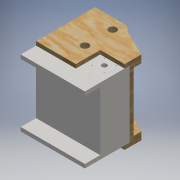
# Autodesk Inventor part: sideskirt_mount
Saved by Autodesk Inventor 2016 SP2 (Build 200236200, 236)
## iProperties
Created: 2017-08-25
Part Number: sideskirt_mount
Material: Generic
Document SubType Name: Modeling
Designer: Admin
Density: 1 g/cm^3
Appearance: Default
Tebal_papan: 15,000 mm
Lebar_base: 230,000 mm
box_nema23: 100,000 mm
d55: 145,251 mm
d60: 230,000 mm
d67: 100,000 mm
d70: 85,000 mm
d73: 230,000 mm
d80: 250,000 mm
d87: 230,000 mm
d94: 230,000 mm
d100: 70,000 mm
d106: 100,000 mm
d110: 230,000 mm
d113: 100,000 mm
d126: 360,00 deg
d0: 30,000 mm
d1: 30,000 mm
d2: 108,000 mm
d3: 150,000 mm
d5: 80,000 mm
d7: 15,000 mm
d8: 0,00 deg
d9: 15,000 mm
d10: 100,000 mm
d11: 100,000 mm
d12: 60,000 mm
d13: 15,000 mm
d14: 0,00 deg
d15: 230,000 mm
d16: 0,00 deg
d17: 80,000 mm
d32: 15,000 mm
d33: 15,000 mm
d34: 15,000 mm
d35: 230,000 mm
d36: 0,00 deg
d37: 230,000 mm
d38: 0,00 deg
d39: 230,000 mm
d40: 0,00 deg
d41: 15,000 mm
d42: 0,00 deg
d43: 15,000 mm
d44: 230,000 mm
d45: 0,00 deg
d46: 15,000 mm
d47: 230,000 mm
d48: 0,00 deg
d52: 15,000 mm
d53: 230,000 mm
d54: 0,00 deg
d56: 48,417 mm
d57: 48,417 mm
d58: 15,000 mm
d59: 0,00 deg
d61: 46,000 mm
d62: 46,000 mm
d63: 46,000 mm
d64: 46,000 mm
d65: 15,000 mm
d66: 0,00 deg
d68: 33,333 mm
d69: 33,333 mm
d71: 15,000 mm
d72: 42,500 mm
d74: 46,000 mm
d75: 46,000 mm
d76: 46,000 mm
d77: 46,000 mm
d78: 15,000 mm
d79: 0,00 deg
d81: 50,000 mm
d82: 50,000 mm
d83: 50,000 mm
d84: 50,000 mm
d85: 15,000 mm
d86: 0,00 deg
d88: 46,000 mm
d89: 46,000 mm
d90: 46,000 mm
d91: 46,000 mm
d92: 15,000 mm
d93: 0,00 deg
d95: 46,000 mm
d96: 46,000 mm
d97: 46,000 mm
d98: 46,000 mm
d99: 15,000 mm
d101: 23,333 mm
d102: 23,333 mm
d103: 15,000 mm
d104: 0,00 deg
d105: 15,000 mm
d107: 33,333 mm
d108: 33,333 mm
d109: 15,000 mm
d111: 32,857 mm
d112: 32,857 mm
d114: 33,333 mm
d115: 15,000 mm
d116: 0,00 deg
d117: 15,000 mm
d118: 15,000 mm
d120: 15,000 mm
d121: 0,00 deg
d122: 4,000 mm
d123: 23,570 mm
d124: 4,000 ul
d128: 20,000 mm
d129: 15,000 mm
d130: 0,00 deg
d131: 15,000 mm
d132: 250,000 mm
d133: 140,000 mm
d134: 95,000 mm
d135: 95,000 mm
Author: Admin
Autodesk Inventor part; units mm, degrees
ref_plane "YZ Plane" through (0, 0, 0) normal (1, 0, 0) x (0, 1, 0)
ref_plane "XZ Plane" through (0, 0, 0) normal (0, 1, 0) x (-1, 0, 0)
sketch "Sketch1" plane through (0, 0, 0) normal (0, 0, 1) x (1, 0, 0)
  circle A0 centre (0, 108) radius 15
  circle A1 centre (0, 0) radius 15
  line L0 (-110, 0) -> (-110, 150)
  line L1 (-110, 150) -> (0, 150)
  line L2 (140, 0) -> (140, -80)
  line L3 (140, -80) -> (0, -80)
  line L4 (-110, 0) -> (-110, -80)
  line L5 (-110, -80) -> (0, -80)
  circle A2 centre (0, 108) radius 42 construction
  arc A3 (35.2506, 130.834) -> (0, 150) centre (0, 108) ccw
  line L6 (140, 0) -> (140, 80)
  line L7 (35.2506, 130.834) -> (140, 80)
  dimension "d0" = 30
  dimension "d1" = 30
  dimension "d2" = 108
  dimension "d3" = 150
  dimension "d5" = 80
  dimension "d17" = 80
  dimension "d132" = 250
  dimension "d133" = 140
  constraints: 16 end point, 5 vertical alignment, 4 centre point, 4 point on circle, 4 vertical, 3 coincident, 3 perpendicular, 2 horizontal alignment
  measures "d0" diameter of A1
  measures "d1" diameter of A0
  measures "d2" distance of point (0, 0) A0.centre
  measures "d3" distance of L0.start L0.end
  measures "d5" distance of L2.start L2.end
  measures "d17" distance of L2.start L6.end
  measures "d132" distance of L4.end L2.end
  measures "d133" distance of L2.start point (0, 0)
extrude "Extrusion1" add sketch "Sketch1" along normal blind 15
sketch "Sketch2" plane through (0, 0, 15) normal (0, 0, 1) x (1, 0, 0)
  line L0 (140, -80) -> (140, 80.0243)
  line L1 (-110, 150) -> (-110, -80) projected
  line L2 (140, -65) -> (-110, -65)
  line L3 (-110, -65) -> (-110, -80)
  line L4 (-110, -80) -> (140, -80)
  line L5 (140, -80) -> (140, -65)
  line L6 (140, -65) -> (40, -65)
  line L7 (40, -65) -> (40, 35)
  line L8 (40, 35) -> (140, 35)
  line L9 (140, 35) -> (140, -65)
  line L10 (140, -80) -> (-110, -80) projected
  line L11 (140, -80) -> (-110, -80)
  line L12 (-110, -80) -> (-110, -140)
  line L13 (-110, -140) -> (140, -140)
  line L14 (140, -140) -> (140, -80)
  point P0 (0, 0)
  point P1 (120, 0)
  dimension "d9" = 15
  dimension "d10" = 100
  dimension "d11" = 100
  dimension "d12" = 60
  constraints: 24 end point, 5 parallel, 3 horizontal, 3 perpendicular, 2 vertical alignment, 1 vertical, 4 other
  measures "d9" distance of L1.end L2.end
  measures "d10" distance of L7.end L8.end
  measures "d11" distance of L6.end L7.end
  measures "d12" distance of L12.end L11.end
extrude "Extrusion2" add sketch "Sketch2" along normal blind 15 separate body
sketch "Sketch3" plane through (0, 0, 30) normal (0, 0, 1) x (1, 0, 0)
  line L0 (40, -65) -> (-110, -65) projected
  line L1 (-110, -80) -> (140, -80) projected
  line L2 (-110, -65) -> (140, -65)
  line L3 (140, -65) -> (140, -80)
  line L4 (140, -80) -> (-110, -80)
  line L5 (-110, -80) -> (-110, -65)
  point P0 (0, 0)
  constraints: 8 end point, 2 parallel, 1 horizontal, 1 perpendicular
extrude "Extrusion3" add sketch "Sketch3" along normal blind 230 separate body
sketch "Sketch5" plane through (0, 0, 30) normal (0, 0, 1) x (1, 0, 0)
  line L0 (40, 35) -> (40, -65) projected
  line L1 (140, 35) -> (40, 35) projected
  line L2 (140, -65) -> (-110, -65) projected
  line L3 (40, 35) -> (55, 35)
  line L4 (55, 35) -> (55, -65)
  line L5 (55, -65) -> (40, -65)
  line L6 (40, -65) -> (40, 35)
  point P0 (0, 0)
  dimension "d32" = 15
  constraints: 8 end point, 2 parallel, 1 horizontal, 1 perpendicular, 1 point on line
  measures "d32" distance of L4.end L5.end
sketch "Sketch6" plane through (0, 0, 30) normal (0, 0, 1) x (1, 0, 0)
  line L0 (140, -140) -> (140, 35) projected
  line L1 (140, 35) -> (40, 35) projected
  line L2 (140, -65) -> (-110, -65) projected
  line L3 (140, 35) -> (125, 35)
  line L4 (125, 35) -> (125, -65)
  line L5 (125, -65) -> (140, -65)
  line L6 (140, -65) -> (140, 35)
  point P0 (0, 0)
  dimension "d33" = 15
  constraints: 8 end point, 2 parallel, 1 horizontal, 1 perpendicular, 1 point on line
  measures "d33" distance of L5.end L4.end
sketch "Sketch7" plane through (0, 0, 30) normal (0, 0, 1) x (1, 0, 0)
  line L0 (140, 35) -> (40, 35) projected
  line L1 (55, 35) -> (125, 35)
  line L2 (55, 20) -> (125, 20)
  line L3 (55, 20) -> (55, 35)
  line L4 (125, 20) -> (125, 35)
  point P0 (0, 0)
  dimension "d34" = 15
  dimension "d117" = 15
  dimension "d118" = 15
  constraints: 8 end point, 2 point on line, 1 horizontal, 1 perpendicular, 1 vertical
  measures "d34" distance between parallel lines of L0 L2
  measures "d117" distance from line of L0.end L3
  measures "d118" distance of L0.start L1.end
extrude "Extrusion8" add sketch "Sketch5" along normal blind 230 separate body
extrude "Extrusion9" add sketch "Sketch7" along normal blind 230 separate body
extrude "Extrusion10" add sketch "Sketch6" along normal blind 230 separate body
sketch "Sketch8" plane through (0, 0, 15) normal (0, 0, 1) x (1, 0, 0)
  circle A0 centre (0, 0) radius 15 projected
  circle A1 centre (0, 108) radius 15 projected
  line L0 (-110, 150) -> (-110, -80) projected
  line L1 (-110, -80) -> (140, -80) projected
  line L2 (140, -80) -> (140, 80) projected
  line L3 (140, 80) -> (35.2506, 130.834) projected
  arc A2 (35.2506, 130.834) -> (0, 150) centre (0, 108) ccw projected
  line L4 (0, 150) -> (-110, 150) projected
  line L5 (125, 35) -> (55, 35) projected
  line L6 (140, 35) -> (125, 35) projected
  line L7 (55, 35) -> (40, 35) projected
  line L8 (40, 35) -> (40, -65) projected
  line L9 (40, -65) -> (-110, -65) projected
  line L10 (-110, 150) -> (-110, -80) projected
  line L11 (-110, 150) -> (-110, -65)
  line L12 (140, 35) -> (40, 35) projected
  line L13 (40, -65) -> (40, 35)
  line L14 (140, -140) -> (140, 35) projected
  line L15 (40, 35) -> (140, 35)
  constraints: 6 end point, 2 perpendicular, 1 vertical
extrude "Extrusion11" add sketch "Sketch8" along normal blind 15 separate body contours L4 A2 L3 L2 L6 L5 L7 L8 L9 L0
sketch "Sketch9" plane through (0, 0, 30) normal (0, 0, 1) x (1, 0, 0)
  line L0 (140, 35) -> (40, 35) projected
  line L1 (140, -80) -> (140, 80) projected
  line L2 (40, 35) -> (140, 35)
  line L3 (140, 35) -> (140, 50)
  line L4 (140, 50) -> (40, 50)
  line L5 (40, 50) -> (40, 35)
  point P0 (0, 0)
  dimension "d43" = 15
  constraints: 8 end point, 2 parallel, 1 horizontal, 1 perpendicular, 1 point on line
  measures "d43" distance of L3.end L2.end
extrude "Extrusion12" add sketch "Sketch9" along normal blind 230 separate body
sketch "Sketch10" plane through (0, 0, 30) normal (0, 0, 1) x (1, 0, 0)
  line L0 (140, -65) -> (-110, -65) projected
  line L1 (40, 35) -> (40, -65) projected
  line L2 (-110, -65) -> (40, -65)
  line L3 (40, -65) -> (40, -50)
  line L4 (40, -50) -> (-110, -50)
  line L5 (-110, -50) -> (-110, -65)
  point P0 (0, 0)
  dimension "d46" = 15
  constraints: 8 end point, 2 parallel, 1 horizontal, 1 perpendicular, 1 point on line
  measures "d46" distance of L3.end L2.end
extrude "Extrusion13" add sketch "Sketch10" along normal blind 230 separate body
sketch "Sketch12" plane through (0, 0, 30) normal (0, 0, 1) x (1, 0, 0)
  line L0 (140, 50) -> (40, 50) projected
  line L1 (40, -50) -> (-110, -50) projected
  line L2 (40, 50) -> (25, 50)
  line L3 (25, 50) -> (25, -50)
  line L4 (25, -50) -> (40, -50)
  line L5 (40, -50) -> (40, 50)
  point P0 (0, 0)
  dimension "d52" = 15
  constraints: 8 end point, 2 parallel, 1 horizontal, 1 perpendicular, 1 point on line
  measures "d52" distance of L4.end L3.end
extrude "Extrusion15" add sketch "Sketch12" along normal blind 230 separate body
sketch "Sketch13" plane through (-110, -50, 30) normal (0, 1, 0) x (1, 0, 0)
  line L0 (110, 0) -> (0, 0) projected
  line L1 (110, 0) -> (145.2506, 0) projected
  line L2 (0, 0) -> (250, 0) projected
  line L3 (150, 15) -> (0, 15) projected
  line L4 (0, 0) -> (48.4169, 0)
  line L5 (48.4169, 0) -> (48.4169, 15)
  line L6 (48.4169, 15) -> (0, 15)
  line L7 (0, 15) -> (0, 0)
  line L8 (145.2506, 0) -> (96.8338, 0)
  line L9 (96.8338, 0) -> (96.8338, 15)
  line L10 (96.8338, 15) -> (145.2506, 15)
  line L11 (145.2506, 15) -> (145.2506, 0)
  line L12 (0, 0) -> (0, -230) projected
  line L13 (0, 0) -> (0, -230) construction
  line L14 (0, -115) -> (68.0794, -115) construction
  line L15 (110, -230) -> (0, -230)
  line L16 (110, -230) -> (145.2506, -230)
  line L17 (150, -245) -> (0, -245)
  line L18 (0, -230) -> (48.4169, -230)
  line L19 (48.4169, -230) -> (48.4169, -245)
  line L20 (48.4169, -245) -> (0, -245)
  line L21 (0, -245) -> (0, -230)
  line L22 (145.2506, -230) -> (96.8338, -230)
  line L23 (96.8338, -230) -> (96.8338, -245)
  line L24 (96.8338, -245) -> (145.2506, -245)
  line L25 (145.2506, -245) -> (145.2506, -230)
  point P0 (110, 30)
  point P1 (110, -260)
  dimension "d55" = 145.2506
  dimension "d56" = 48.4169
  dimension "d57" = 48.4169
  constraints: 40 end point, 11 symmetric about line, 4 parallel, 4 point on line, 3 horizontal, 2 perpendicular, 1 midpoint
  measures "d55" distance of L1.end L0.end
  measures "d56" distance of L3.end L5.end
  measures "d57" distance of L10.end L9.end
extrude "Extrusion16" add sketch "Sketch13" against normal blind 15 contours L0 L9 L3 L11 L1 | L0 L7 L3 L5 | L16 L25 L17 L23 L15 | L19 L17 L21 L15 bodies 9
sketch "Sketch14" plane through (40, 50, 30) normal (0, 1, 0) x (1, 0, 0)
  line L0 (0, 0) -> (0, -230) projected
  line L1 (100, -230) -> (0, -230) projected
  line L2 (50, -230) -> (50, -65.4779) construction
  line L3 (-15, 0) -> (-15, -230) projected
  line L4 (0, 0) -> (-15, 0)
  line L5 (-15, 0) -> (-15, -46)
  line L6 (-15, -46) -> (0, -46)
  line L7 (0, -46) -> (0, 0)
  line L8 (0, 0) -> (0, -230) projected
  line L9 (0, -92) -> (-15, -92)
  line L10 (-15, -92) -> (-15, -138)
  line L11 (-15, -138) -> (0, -138)
  line L12 (0, -138) -> (0, -92)
  line L13 (0, -230) -> (-15, -230) projected
  line L14 (0, -230) -> (-15, -230)
  line L15 (-15, -230) -> (-15, -184)
  line L16 (-15, -184) -> (0, -184)
  line L17 (0, -184) -> (0, -230)
  line L18 (100, 15) -> (0, 15) projected
  line L19 (0, 0) -> (33.3333, 0)
  line L20 (33.3333, 0) -> (33.3333, 15)
  line L21 (33.3333, 15) -> (0, 15)
  line L22 (0, 15) -> (0, 0)
  line L23 (100, 0) -> (0, 0) projected
  line L24 (66.6667, 0) -> (100, 0)
  line L25 (100, 0) -> (100, 15)
  line L26 (100, 15) -> (66.6667, 15)
  line L27 (66.6667, 15) -> (66.6667, 0)
  line L28 (0, -115) -> (60, -115) construction
  line L29 (0, -230) -> (33.3333, -230)
  line L30 (33.3333, -230) -> (33.3333, -245)
  line L31 (33.3333, -245) -> (0, -245)
  line L32 (0, -245) -> (0, -230)
  line L33 (66.6667, -230) -> (100, -230)
  line L34 (100, -230) -> (100, -245)
  line L35 (100, -245) -> (66.6667, -245)
  line L36 (66.6667, -245) -> (66.6667, -230)
  point P0 (-40, 30)
  dimension "d60" = 230
  dimension "d61" = 46
  dimension "d62" = 46
  dimension "d63" = 46
  dimension "d64" = 46
  dimension "d67" = 100
  dimension "d68" = 33.3333
  dimension "d69" = 33.3333
  constraints: 60 end point, 10 parallel, 9 symmetric about line, 6 perpendicular, 6 point on line, 5 horizontal, 2 midpoint, 1 vertical
  measures "d60" distance of L0.end L0.start
  measures "d61" distance of L5.end L3.start
  measures "d62" distance of L9.end L5.end
  measures "d63" distance of L10.end L9.end
  measures "d64" distance of L3.end L15.end
  measures "d67" distance of L1.start L0.end
  measures "d68" distance of L20.end L18.end
  measures "d69" distance of L18.start L26.end
extrude "Extrusion17" add sketch "Sketch14" against normal blind 15 contours L1 L30 L31 L32 | L0 L6 L3 L4 | L22 L18 L20 L19 | L0 L11 L3 L9 | L27 L18 L25 L23 | L0 L13 L3 L16 | L34 L35 L36 L1 bodies 8
sketch "Sketch15" plane through (25, -50, 30) normal (-1, 0, 0) x (0, 0, 1)
  line L0 (230, 85) -> (184, 85) projected
  line L1 (230, 100) -> (230, 0) projected
  line L2 (230, 85) -> (245, 85)
  line L3 (245, 85) -> (245, 42.5)
  line L4 (245, 42.5) -> (230, 42.5)
  line L5 (230, 42.5) -> (230, 85)
  line L6 (0, 100) -> (230, 100) construction
  line L7 (115, 100) -> (115, 19.3986) construction
  line L8 (0, 85) -> (-15, 85)
  line L9 (-15, 85) -> (-15, 42.5)
  line L10 (-15, 42.5) -> (0, 42.5)
  line L11 (0, 42.5) -> (0, 85)
  line L12 (0, 0) -> (230, 0) construction
  line L13 (0, -15) -> (230, -15) projected
  line L14 (184, 0) -> (138, 0)
  line L15 (138, 0) -> (138, -15)
  line L16 (138, -15) -> (184, -15)
  line L17 (184, -15) -> (184, 0)
  line L18 (92, 0) -> (46, 0)
  line L19 (46, 0) -> (46, -15)
  line L20 (46, -15) -> (92, -15)
  line L21 (92, -15) -> (92, 0)
  point P0 (-30, 50)
  dimension "d70" = 85
  dimension "d71" = 15
  dimension "d72" = 42.5
  dimension "d73" = 230
  dimension "d74" = 46
  dimension "d75" = 46
  dimension "d76" = 46
  dimension "d77" = 46
  constraints: 34 end point, 6 parallel, 4 point on line, 4 symmetric about line, 3 horizontal, 3 perpendicular, 1 midpoint, 1 vertical
  measures "d70" distance of L1.end L0.start
  measures "d71" distance of L3.end L4.end
  measures "d72" distance of L2.end L3.end
  measures "d73" distance of L12.start L1.end
  measures "d74" distance of L14.end L14.start
  measures "d75" distance of L1.end L14.start
  measures "d76" distance of L18.start L14.end
  measures "d77" distance of L18.end L18.start
extrude "Extrusion18" add sketch "Sketch15" against normal blind 15 bodies 10
combine bodies "Combine1" operation type subtract main body 10 bodies to subtract 8 keep tools yes
combine bodies "Combine2" operation type subtract main body 9 bodies to subtract 10 keep tools yes
sketch "Sketch16" plane through (-110, -65, 30) normal (0, 1, 0) x (1, 0, 0)
  line L0 (0, 0) -> (0, -230) projected
  line L1 (250, 0) -> (250, -230) projected
  line L2 (250, 0) -> (235, 0) projected
  line L3 (250, 15) -> (150, 15) projected
  line L4 (250, 0) -> (200, 0)
  line L5 (200, 0) -> (200, 15)
  line L6 (200, 15) -> (250, 15)
  line L7 (250, 15) -> (250, 0)
  line L8 (250, 0) -> (150, 0) projected
  line L9 (150, 15) -> (0, 15) projected
  line L10 (150, 0) -> (100, 0)
  line L11 (100, 0) -> (100, 15)
  line L12 (100, 15) -> (150, 15)
  line L13 (150, 15) -> (150, 0)
  line L14 (50, 0) -> (0, 0)
  line L15 (0, 0) -> (0, 15)
  line L16 (0, 15) -> (50, 15)
  line L17 (50, 15) -> (50, 0)
  line L18 (0, -115) -> (76.9217, -115) construction
  line L19 (250, -230) -> (235, -230)
  line L20 (250, -245) -> (150, -245)
  line L21 (250, -230) -> (200, -230)
  line L22 (200, -230) -> (200, -245)
  line L23 (200, -245) -> (250, -245)
  line L24 (250, -245) -> (250, -230)
  line L25 (250, -230) -> (150, -230)
  line L26 (150, -245) -> (0, -245)
  line L27 (150, -230) -> (100, -230)
  line L28 (100, -230) -> (100, -245)
  line L29 (100, -245) -> (150, -245)
  line L30 (150, -245) -> (150, -230)
  line L31 (50, -230) -> (0, -230)
  line L32 (0, -230) -> (0, -245)
  line L33 (0, -245) -> (50, -245)
  line L34 (50, -245) -> (50, -230)
  point P0 (110, 30)
  dimension "d80" = 250
  dimension "d81" = 50
  dimension "d82" = 50
  dimension "d83" = 50
  dimension "d84" = 50
  constraints: 58 end point, 16 symmetric about line, 6 parallel, 6 point on line, 4 horizontal, 3 midpoint, 3 perpendicular
  measures "d80" distance between parallel lines of L0 L1
  measures "d81" distance of L9.end L16.end
  measures "d82" distance of L16.end L11.end
  measures "d83" distance from line of L13 L11.end
  measures "d84" distance from line of L5 L3.start
extrude "Extrusion19" add sketch "Sketch16" against normal blind 15 contours L15 L9 L17 L14 | L31 L34 L26 L32 | L9 L13 L10 L11 | L28 L27 L30 L26 | L3 L7 L2 L4 L5 | L22 L21 L19 L24 L20 bodies 3
sketch "Sketch17" plane through (40, -65, 30) normal (-1, 0, 0) x (0, 0, 1)
  line L0 (-15, 0) -> (245, 0) projected
  line L1 (0, 0) -> (230, 0) projected
  line L2 (-15, -15) -> (245, -15) projected
  line L3 (46, 0) -> (92, 0)
  line L4 (92, 0) -> (92, -15)
  line L5 (92, -15) -> (46, -15)
  line L6 (46, -15) -> (46, 0)
  line L7 (138, 0) -> (184, 0)
  line L8 (184, 0) -> (184, -15)
  line L9 (184, -15) -> (138, -15)
  line L10 (138, -15) -> (138, 0)
  line L11 (230, 100) -> (230, 0) projected
  line L12 (0, 100) -> (0, 0) projected
  line L13 (0, 66.6667) -> (-15, 66.6667)
  line L14 (-15, 66.6667) -> (-15, 33.3333)
  line L15 (-15, 33.3333) -> (0, 33.3333)
  line L16 (0, 33.3333) -> (0, 66.6667)
  line L17 (0, 0) -> (230, 0) construction
  line L18 (115, 0) -> (115, 50.3337) construction
  line L19 (230, 66.6667) -> (245, 66.6667)
  line L20 (245, 66.6667) -> (245, 33.3333)
  line L21 (245, 33.3333) -> (230, 33.3333)
  line L22 (230, 33.3333) -> (230, 66.6667)
  point P0 (-30, 65)
  dimension "d87" = 230
  dimension "d88" = 46
  dimension "d89" = 46
  dimension "d90" = 46
  dimension "d91" = 46
  dimension "d105" = 15
  dimension "d106" = 100
  dimension "d107" = 33.3333
  dimension "d108" = 33.3333
  constraints: 34 end point, 6 parallel, 5 point on line, 4 symmetric about line, 3 horizontal, 3 perpendicular, 1 midpoint, 1 vertical
  measures "d87" distance between parallel lines of L11 L12
  measures "d88" distance from line of L4 L5.end
  measures "d89" distance of L4.end L9.end
  measures "d90" distance between parallel lines of L8 L10
  measures "d91" distance between parallel lines of L12 L6
  measures "d105" distance of L13.end L13.start
  measures "d106" distance of L1.start L12.start
  measures "d107" vertical distance of L12.start L13.end
  measures "d108" distance of L14.end L13.end
extrude "Extrusion20" add sketch "Sketch17" against normal blind 15 contours L0 L4 L2 L6 | L0 L8 L2 L10 | L19 L20 L21 L11 | L12 L15 L14 L13 bodies 4
sketch "Sketch18" plane through (55, 35, 30) normal (0, 1, 0) x (1, 0, 0)
  line L0 (70, 0) -> (70, -230) projected
  line L1 (0, 0) -> (0, -230) projected
  line L2 (70, 0) -> (70, -230) projected
  line L3 (85, 0) -> (85, -230) projected
  line L4 (70, -46) -> (85, -46)
  line L5 (85, -46) -> (85, -92)
  line L6 (85, -92) -> (70, -92)
  line L7 (70, -92) -> (70, -46)
  line L8 (70, -138) -> (85, -138)
  line L9 (85, -138) -> (85, -184)
  line L10 (85, -184) -> (70, -184)
  line L11 (70, -184) -> (70, -138)
  line L12 (0, 0) -> (70, 0) construction
  line L13 (35, 0) -> (35, -84.66) construction
  line L14 (0, -46) -> (-15, -46)
  line L15 (-15, -46) -> (-15, -92)
  line L16 (-15, -92) -> (0, -92)
  line L17 (0, -92) -> (0, -46)
  line L18 (0, -138) -> (-15, -138)
  line L19 (-15, -138) -> (-15, -184)
  line L20 (-15, -184) -> (0, -184)
  line L21 (0, -184) -> (0, -138)
  line L22 (46.6667, 0) -> (23.3333, 0)
  line L23 (23.3333, 0) -> (23.3333, 15)
  line L24 (23.3333, 15) -> (46.6667, 15)
  line L25 (46.6667, 15) -> (46.6667, 0)
  line L26 (70, -115) -> (29.7795, -115) construction
  line L27 (46.6667, -230) -> (23.3333, -230)
  line L28 (23.3333, -230) -> (23.3333, -245)
  line L29 (23.3333, -245) -> (46.6667, -245)
  line L30 (46.6667, -245) -> (46.6667, -230)
  point P0 (-55, 30)
  point P1 (35, -230)
  dimension "d94" = 230
  dimension "d95" = 46
  dimension "d96" = 46
  dimension "d97" = 46
  dimension "d98" = 46
  dimension "d99" = 15
  dimension "d100" = 70
  dimension "d101" = 23.3333
  dimension "d102" = 23.3333
  constraints: 52 end point, 13 symmetric about line, 6 parallel, 5 point on line, 4 horizontal, 3 perpendicular, 2 midpoint, 1 vertical
  measures "d94" distance of L0.end L0.start
  measures "d95" distance of L5.end L4.end
  measures "d96" distance of L3.start L4.end
  measures "d97" distance of L8.end L5.end
  measures "d98" distance of L9.end L8.end
  measures "d99" distance of L24.end L22.start
  measures "d100" distance of L1.start L2.start
  measures "d101" distance of L23.end L24.end
  measures "d102" distance of L2.start L22.start
extrude "Extrusion21" add sketch "Sketch18" against normal blind 15 contours L4 L3 L6 L0 | L8 L3 L10 L0 | L1 L16 L15 L14 | L1 L20 L19 L18 | L22 L23 L24 L25 | L30 L29 L28 L27 bodies 5
sketch "Sketch19" plane through (140, -65, 30) normal (1, 0, 0) x (0, 0, -1)
  line L0 (0, 0) -> (-230, 0) projected
  line L1 (-197.1429, 0) -> (-164.2857, 0)
  line L2 (-164.2857, 0) -> (-164.2857, -15)
  line L3 (-164.2857, -15) -> (-197.1429, -15)
  line L4 (-197.1429, -15) -> (-197.1429, 0)
  line L5 (-230, 100) -> (-230, 66.6667) projected
  line L6 (-230, 66.6667) -> (-245, 66.6667)
  line L7 (-245, 66.6667) -> (-245, 33.3333)
  line L8 (-245, 33.3333) -> (-230, 33.3333)
  line L9 (-230, 33.3333) -> (-230, 66.6667)
  line L10 (0, 0) -> (-230, 0) construction
  line L11 (-115, 0) -> (-115, 58.0259) construction
  line L12 (0, 66.6667) -> (15, 66.6667)
  line L13 (15, 66.6667) -> (15, 33.3333)
  line L14 (15, 33.3333) -> (0, 33.3333)
  line L15 (0, 33.3333) -> (0, 66.6667)
  line L16 (-245, -15) -> (15, -15) projected
  line L17 (-65.7143, 0) -> (-32.8571, 0)
  line L18 (-32.8571, 0) -> (-32.8571, -15)
  line L19 (-32.8571, -15) -> (-65.7143, -15)
  line L20 (-65.7143, -15) -> (-65.7143, 0)
  point P0 (30, 65)
  dimension "d109" = 15
  dimension "d110" = 230
  dimension "d111" = 32.8571
  dimension "d112" = 32.8571
  dimension "d113" = 100
  dimension "d114" = 33.3333
  dimension "d131" = 15
  dimension "d136" = 32.8571
  dimension "d138" = 32.8571
  constraints: 34 end point, 6 parallel, 4 symmetric about line, 3 horizontal, 3 perpendicular, 3 point on line, 1 midpoint, 1 vertical
  measures "d109" distance of L1.end L2.end
  measures "d110" distance of L0.start L0.end
  measures "d111" horizontal distance of L0.end L3.end
  measures "d112" distance of L3.end L2.end
  measures "d113" distance of L0.end L5.start
  measures "d114" distance of L7.end L6.end
  measures "d131" distance of L5.end L6.end
  measures "d136" distance of L18.end L19.end
  measures "d138" horizontal distance of L18.end L0.start
extrude "Extrusion22" add sketch "Sketch19" against normal blind 15 contours L18 L16 L20 L0 | L2 L3 L4 L0 | L9 L8 L7 L6 | L12 L13 L14 L15 bodies 6
combine bodies "Combine3" operation type subtract main body 6 bodies to subtract 5 keep tools yes
combine bodies "Combine4" operation type subtract main body 4 bodies to subtract 5 keep tools yes
combine bodies "Combine5" operation type subtract main body 7 bodies to subtract 9 keep tools yes
combine bodies "Combine6" operation type subtract main body 7 bodies to subtract 10 keep tools yes
combine bodies "Combine7" operation type subtract main body 7 bodies to subtract 8 keep tools yes
combine bodies "Combine8" operation type subtract main body 2 bodies to subtract 6 keep tools yes
combine bodies "Combine9" operation type subtract main body 2 bodies to subtract 5 keep tools yes
combine bodies "Combine10" operation type subtract main body 2 bodies to subtract 4 keep tools yes
ref_plane "Work Plane1" through (-110, -65, 145) normal (0, 0, 1) x (1, 0, 0)
combine bodies "Combine11" operation type subtract main body 2 bodies to subtract 3 keep tools yes
sketch "Sketch22" plane through (0, 0, 15) normal (0, 0, -1) x (-1, 0, 0)
  line L0 (-55, 20) -> (-78.3333, 20) construction
  line L1 (-125, 20) -> (-55, 20) construction
  line L2 (-55, 20) -> (-55, -48.3333) construction
  line L3 (-55, -65) -> (-55, -31.6667) construction
  line L4 (-125, -48.3333) -> (-125, 20) construction
  line L5 (-125, 35) -> (-125, 1.6667) construction
  line L6 (-125, -48.3333) -> (-55, -48.3333) construction
  line L7 (-125, -31.6667) -> (-125, -65) construction
  line L8 (-125, 20) -> (-55, -48.3333) construction
  line L9 (-125, -31.6667) -> (-125, 1.6667) construction
  line L10 (-125, -15) -> (-55, -14.1667) construction
  circle A0 centre (-113.434, 8.7094) radius 2
  line L11 (-78.3333, 20) -> (-101.6667, 20) construction
  line L12 (-90, 20) -> (-90, -48.3333) construction
  circle A1 centre (-112.876, -37.6006) radius 2
  circle A2 centre (-66.566, -37.0427) radius 2
  circle A3 centre (-67.124, 9.2673) radius 2
  circle A4 centre (-90, -14.1667) radius 10
  point P0 (0, 0)
  dimension "d122" = 4
  dimension "d123" = 23.57
  dimension "d126" = 360
  dimension "d128" = 20
  constraints: 14 end point, 6 midpoint, 5 centre point, 2 collinear, 1 coincident, 1 perpendicular, 1 point on line, 9 other
  measures "d122" diameter of A0
  measures "d123" distance from line of L10 A0.centre
  measures "d128" diameter of A4
extrude "Extrusion24" cut sketch "Sketch22" against normal blind 15 bodies 2
mirror "Mirror1" about plane through (-110, -65, 145) normal (0, 0, 1) bodies 2
mirror "Mirror2" about plane through (-110, -65, 145) normal (0, 0, 1) bodies 7
sketch "Sketch20" plane through (0, 0, 0) normal (0, 0, -1) x (-1, 0, 0)
  line L0 (-140, -140) -> (-140, -80) projected
  line L1 (-140, -80) -> (-45, -80)
  line L2 (-45, -80) -> (-45, 15)
  line L3 (-45, 15) -> (-140, 15)
  line L4 (-140, 15) -> (-140, -80)
  point P0 (0, 0)
  point P1 (-110, -65)
  dimension "d134" = 95
  dimension "d135" = 95
  constraints: 8 end point, 2 parallel, 1 horizontal, 1 perpendicular, 1 other
  measures "d134" distance of L3.end L1.start
  measures "d135" distance of L1.start L1.end
extrude "Extrusion23" cut sketch "Sketch20" against normal blind 15 bodies 1
mirror "Mirror3" about plane through (-110, -65, 145) normal (0, 0, 1) bodies 1
combine bodies "Combine12" operation type subtract main body 3 bodies to subtract 6 keep tools yes
combine bodies "Combine13" operation type subtract main body 3 bodies to subtract 4 keep tools yes
equation "\"d7\" = Tebal_papan"
equation "\"d9\" = Tebal_papan"
equation "\"d10\" = box_nema23"
equation "\"d11\" = box_nema23"
equation "\"d13\" = Tebal_papan"
equation "\"d15\" = Lebar_base"
equation "\"d32\" = Tebal_papan"
equation "\"d33\" = Tebal_papan"
equation "\"d34\" = Tebal_papan"
equation "\"d117\" = Tebal_papan"
equation "\"d118\" = Tebal_papan"
equation "\"d35\" = Lebar_base"
equation "\"d37\" = Lebar_base"
equation "\"d39\" = Lebar_base"
equation "\"d41\" = Tebal_papan"
equation "\"d43\" = Tebal_papan"
equation "\"d44\" = Lebar_base"
equation "\"d46\" = Tebal_papan"
equation "\"d47\" = Lebar_base"
equation "\"d52\" = Tebal_papan"
equation "\"d53\" = Lebar_base"
equation "\"d56\" = 0.333333 * d55"
equation "\"d57\" = d56"
equation "\"d58\" = Tebal_papan"
equation "\"d61\" = 0.2 * d60"
equation "\"d62\" = d61"
equation "\"d63\" = d62"
equation "\"d64\" = d63"
equation "\"d68\" = 0.333333 * d67"
equation "\"d69\" = d68"
equation "\"d65\" = Tebal_papan"
equation "\"d71\" = Tebal_papan"
equation "\"d72\" = 0.5 * d70"
equation "\"d74\" = 0.2 * d73"
equation "\"d75\" = d74"
equation "\"d76\" = d74"
equation "\"d77\" = d76"
equation "\"d78\" = Tebal_papan"
equation "\"d81\" = 0.2 * d80"
equation "\"d82\" = d81"
equation "\"d83\" = d82"
equation "\"d84\" = d82"
equation "\"d85\" = Tebal_papan"
equation "\"d88\" = 0.2 * d87"
equation "\"d89\" = d88"
equation "\"d90\" = d89"
equation "\"d91\" = d88"
equation "\"d105\" = Tebal_papan"
equation "\"d107\" = 0.333333 * d106"
equation "\"d108\" = d107"
equation "\"d92\" = Tebal_papan"
equation "\"d95\" = 0.2 * d94"
equation "\"d96\" = d95"
equation "\"d97\" = d95"
equation "\"d98\" = d95"
equation "\"d99\" = Tebal_papan"
equation "\"d101\" = 0.333333 * d100"
equation "\"d102\" = d101"
equation "\"d103\" = Tebal_papan"
equation "\"d109\" = Tebal_papan"
equation "\"d111\" = 0.142857 * d110"
equation "\"d112\" = d111"
equation "\"d114\" = 0.333333 * d113"
equation "\"d131\" = Tebal_papan"
equation "\"d136\" = d111"
equation "\"d138\" = d111"
equation "\"d115\" = Tebal_papan"
equation "\"d129\" = Tebal_papan"
equation "\"d120\" = Tebal_papan"
equation "\"Tebal_papan\" = 15"
equation "\"Lebar_base\" = 230"
equation "\"box_nema23\" = 100"
